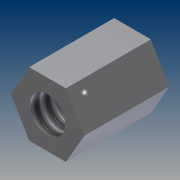
# Autodesk Inventor part: standoffiPart-01
Saved by Autodesk Inventor 2011 SP1 (Build 150282100, 282)
## iProperties
Created: 2011-07-21
Part Number: standoffiPart-01
Document SubType Name: Modeling
Designer: Nathan
Density: 1 g/cm^3
Author: Nathan
Autodesk Inventor part; units mm, degrees
ref_plane "YZ Plane" through (0, 0, 0) normal (1, 0, 0) x (0, 1, 0)
ref_plane "XZ Plane" through (0, 0, 0) normal (0, 1, 0) x (-1, 0, 0)
ref_plane "XY Plane" through (0, 0, 0) normal (0, 0, 1) x (1, 0, 0)
sketch "Sketch1" plane through (0, 0, 0) normal (0, 0, 1) x (1, 0, 0)
  line L0 (2.7496, 0) -> (1.3748, -2.3812)
  line L1 (1.3748, -2.3812) -> (-1.3748, -2.3812)
  line L2 (-1.3748, -2.3812) -> (-2.7496, 0)
  line L3 (-2.7496, 0) -> (-1.3748, 2.3813)
  line L4 (-1.3748, 2.3813) -> (1.3748, 2.3813)
  line L5 (1.3748, 2.3813) -> (2.7496, 0)
  point P0 (0, 0)
  point P1 (0, 0)
  dimension "Diameter" = 4.7625
  constraints: 12 end point, 1 coincident, 13 other
  measures "Diameter" distance between parallel lines of L4 L1
extrude "Extrusion1" add sketch "Sketch1" along normal blind 6.35
sketch "Sketch2" plane through (0, 0, 6.35) normal (0, 0, 1) x (1, 0, 0)
  point P0 (0, 0)
  point P1 (0, 0)
  constraints: 1 coincident
hole "Hole1" at (0, 0, 6.35) direction (0, 0, -1) diameter 2.6416 end through all thread size "6-32 UNC" class "2B" standard "ANSI Unified Screw Threads"
body "Solid1"
